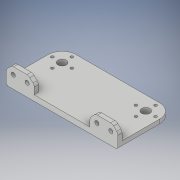
# Autodesk Inventor part: body_v3
Saved by Autodesk Inventor 2019 (Build 230136000, 136)
## iProperties
Created: 2018-12-28
Part Number: body_v3
Material: Generic
Document SubType Name: Modeling
Designer: Daniel
Density: 1 g/cm^3
Appearance: Default
Author: Daniel
Autodesk Inventor part; units mm, degrees
ref_plane "YZ Plane" through (0, 0, 0) normal (1, 0, 0) x (0, 1, 0)
ref_plane "XZ Plane" through (0, 0, 0) normal (0, 1, 0) x (-1, 0, 0)
ref_plane "XY Plane" through (0, 0, 0) normal (0, 0, 1) x (1, 0, 0)
sketch "Sketch1" plane through (0, 0, 0) normal (0, 1, 0) x (-1, 0, 0)
  line L0 (56, 0) -> (-56, 0) projected
  line L1 (0, -49) -> (0, 49) projected
  line L2 (40, -20) -> (-40, -20)
  line L3 (-40, -20) -> (-40, 20)
  line L4 (-40, 20) -> (40, 20)
  line L5 (40, 20) -> (40, -20)
  line L6 (27.5, -35) -> (-27.5, -35) construction
  line L7 (-27.5, -35) -> (-27.5, 35) construction
  line L8 (-27.5, 35) -> (27.5, 35) construction
  line L9 (27.5, 35) -> (27.5, -35) construction
  point P0 (0, 0)
  dimension "d0" = 80
  dimension "d1" = 40
  dimension "d2" = 70
  dimension "d3" = 55
  constraints: 16 end point, 4 parallel, 2 horizontal, 2 perpendicular, 4 other
  measures "d0" distance between parallel lines of L3 L5
  measures "d1" distance between parallel lines of L4 L2
  measures "d2" distance between parallel lines of L8 L6
  measures "d3" distance between parallel lines of L9 L7
extrude "Extrusion1" add sketch "Sketch1" along normal blind 4
sketch "Sketch18" plane through (0, 4, 0) normal (0, 1, 0) x (1, 0, 0)
  line L0 (40, 20) -> (-40, 20) projected
  line L1 (-40, 20) -> (-40, -20) projected
  line L2 (-40, -20) -> (40, -20) projected
  line L3 (40, -20) -> (40, 20) projected
  line L4 (-40, -20) -> (40, -20)
  line L5 (40, -20) -> (40, -17)
  line L6 (40, -17) -> (-40, -17)
  line L7 (-40, -17) -> (-40, -20)
  line L8 (-40, 20) -> (-40, -20) projected
  line L9 (40, -20) -> (40, 20) projected
  line L10 (-40, -20) -> (40, -20) projected
  point P0 (0, 0)
  dimension "d207" = 3
  constraints: 8 end point, 3 collinear, 2 parallel, 1 horizontal, 1 perpendicular
  measures "d207" distance between parallel lines of L6 L4
extrude "Extrusion13" add sketch "Sketch18" along normal blind 10 contours L3 L2 L1 L6
sketch "Sketch19" plane through (0, 4, 0) normal (0, 1, 0) x (1, 0, 0)
  line L0 (-40, -17) -> (40, -17) projected
  line L1 (40, -17) -> (40, 20) projected
  line L2 (40, 20) -> (-40, 20) projected
  line L3 (-40, 20) -> (-40, -17) projected
  line L4 (0, 28) -> (0, -28) projected
  point P0 (0, 0)
  point P1 (-30, 10)
  point P2 (30, 10)
  dimension "d210" = 10
  dimension "d211" = 10
  constraints: 1 symmetric about line
  measures "d210" distance from line of L3 point (-30, 10)
  measures "d211" distance from line of L2 point (-30, 10)
hole "Hole9" at (-30, 4, -10) at (30, 4, -10) direction (0, -1, 0) diameter 6 end through all
sketch "Sketch20" plane through (0, 4, 0) normal (0, 1, 0) x (1, 0, 0)
  circle A0 centre (-30, 10) radius 3 projected
  line L0 (-40, -17) -> (40, -17) projected
  line L1 (40, -17) -> (40, 20) projected
  line L2 (40, 20) -> (-40, 20) projected
  line L3 (-40, 20) -> (-40, -17) projected
  line L4 (-30, -17) -> (-30, 20) construction
  line L5 (-40, 20) -> (-40, -17) projected
  line L6 (40, 20) -> (-40, 20) projected
  line L7 (40, -17) -> (-40, -17) projected
  line L8 (-39.3154, 10) -> (-16.7888, 10) construction
  line L9 (0, 28) -> (0, -28) projected
  point P0 (0, 0)
  point P1 (-37, 10)
  point P2 (-23, 10)
  point P3 (-30, 3)
  point P4 (-30, 17)
  point P5 (37, 10)
  point P6 (23, 10)
  point P7 (30, 3)
  point P8 (30, 17)
  dimension "d219" = 7
  dimension "d220" = 7
  dimension "d221" = 7
  dimension "d222" = 7
  constraints: 8 point on line, 4 end point, 4 symmetric about line, 1 horizontal, 1 parallel, 1 vertical
  measures "d219" distance of A0.centre point (-30, 3)
  measures "d220" distance of A0.centre point (-37, 10)
  measures "d221" distance of A0.centre point (-30, 17)
  measures "d222" distance of A0.centre point (-23, 10)
hole "Hole10" at (-37, 4, -10) at (-23, 4, -10) at (-30, 4, -3) at (-30, 4, -17) at (30, 4, -3) at (37, 4, -10) at (30, 4, -17) at (23, 4, -10) direction (0, -1, 0) diameter 2 end through all
fillet "Fillet11" radius 10 2 edges at (40, 2, -20) (-40, 2, -20)
sketch "Sketch21" plane through (40, 4, 17) normal (0, 0, -1) x (-1, 0, 0)
  line L0 (80, 0) -> (0, 0) projected
  line L1 (80, 0) -> (80, 10) projected
  line L2 (0, 10) -> (80, 10) projected
  line L3 (0, 0) -> (0, 10) projected
  point P0 (40, -4)
  point P1 (5, 5)
  point P2 (75, 5)
  dimension "d232" = 5
  dimension "d233" = 5
  dimension "d234" = 5
  dimension "d235" = 5
  measures "d232" distance from line of L3 point (5, 5)
  measures "d233" distance from line of L2 point (5, 5)
  measures "d234" distance from line of L2 point (75, 5)
  measures "d235" distance from line of L1 point (75, 5)
hole "Hole11" at (35, 9, 17) at (-35, 9, 17) direction (0, 0, 1) diameter 3 end through all
chamfer "Chamfer5" distance 4 angle 45 2 edges at (-40, 14, 18.5) (40, 14, 18.5)
fillet "Fillet12" radius 3 4 edges at (-36, 14, 18.5) (-40, 10, 18.5) (36, 14, 18.5) (40, 10, 18.5)
sketch "Sketch22" plane through (40, 4, 17) normal (0, 0, -1) x (-1, 0, 0)
  circle A0 centre (5, 5) radius 1.5 projected
  circle A1 centre (75, 5) radius 1.5 projected
  arc A2 (0.8787, 6.8787) -> (0, 4.7574) centre (3, 4.7574) ccw projected
  line L0 (0, 0) -> (0, 4.7574) projected
  line L1 (80, 0) -> (0, 0) projected
  line L2 (80, 0) -> (80, 4.7574) projected
  arc A3 (80, 4.7574) -> (79.1213, 6.8787) centre (77, 4.7574) ccw projected
  line L3 (76.8787, 9.1213) -> (79.1213, 6.8787) projected
  arc A4 (76.8787, 9.1213) -> (74.7574, 10) centre (74.7574, 7) ccw projected
  line L4 (5.2426, 10) -> (74.7574, 10) projected
  arc A5 (5.2426, 10) -> (3.1213, 9.1213) centre (5.2426, 7) ccw projected
  line L5 (0.8787, 6.8787) -> (3.1213, 9.1213) projected
  line L6 (10, 0) -> (70, 0) projected
  line L7 (20, 10) -> (60, 10)
  line L8 (60, 10) -> (60, 0)
  line L9 (60, 0) -> (20, 0)
  line L10 (20, 0) -> (20, 10)
  point P0 (40, -4)
  point P1 (40, 5)
  dimension "d247" = 5
  dimension "d248" = 40
  dimension "d256" = 40
  dimension "d257" = 10
  dimension "d258" = 20
  constraints: 8 end point, 2 parallel, 1 horizontal, 1 perpendicular, 1 point on line
  measures "d247" distance from line of L4 point (40, 5)
  measures "d248" distance from line of L0 point (40, 5)
  measures "d256" distance between parallel lines of L8 L10
  measures "d257" distance between parallel lines of L1 L7
  measures "d258" distance between parallel lines of L0 L10
extrude "Extrusion14" cut sketch "Sketch22" against normal up to next contours L4 L8 L1 L10
chamfer "Chamfer6" distance 4 angle 45 2 edges at (-20, 14, 18.5) (20, 14, 18.5)
fillet "Fillet13" radius 3 4 edges at (-24, 14, 18.5) (-20, 10, 18.5) (24, 14, 18.5) (20, 10, 18.5)
sketch "Sketch23" plane through (40, 4, 17) normal (0, 0, -1) x (-1, 0, 0)
  arc A0 (20, 4.7574) -> (19.1213, 6.8787) centre (17, 4.7574) ccw projected
  line L0 (16.8787, 9.1213) -> (19.1213, 6.8787) projected
  arc A1 (16.8787, 9.1213) -> (14.7574, 10) centre (14.7574, 7) ccw projected
  line L1 (5.2426, 10) -> (14.7574, 10) projected
  arc A2 (5.2426, 10) -> (3.1213, 9.1213) centre (5.2426, 7) ccw projected
  line L2 (0.8787, 6.8787) -> (3.1213, 9.1213) projected
  arc A3 (0.8787, 6.8787) -> (0, 4.7574) centre (3, 4.7574) ccw projected
  line L3 (0, 0) -> (0, 4.7574) projected
  line L4 (20, 0) -> (0, 0) projected
  line L5 (20, 0) -> (20, 4.7574) projected
  circle A4 centre (5, 5) radius 1.5 projected
  arc A5 (60.8787, 6.8787) -> (60, 4.7574) centre (63, 4.7574) ccw projected
  line L6 (60, 4.7574) -> (60, 0) projected
  line L7 (80, 0) -> (60, 0) projected
  line L8 (80, 0) -> (80, 4.7574) projected
  arc A6 (80, 4.7574) -> (79.1213, 6.8787) centre (77, 4.7574) ccw projected
  line L9 (76.8787, 9.1213) -> (79.1213, 6.8787) projected
  arc A7 (76.8787, 9.1213) -> (74.7574, 10) centre (74.7574, 7) ccw projected
  line L10 (65.2426, 10) -> (74.7574, 10) projected
  arc A8 (65.2426, 10) -> (63.1213, 9.1213) centre (65.2426, 7) ccw projected
  line L11 (60.8787, 6.8787) -> (63.1213, 9.1213) projected
  circle A9 centre (75, 5) radius 1.5 projected
  point P0 (40, -4)
  point P1 (15, 5)
  point P2 (65, 5)
  dimension "d265" = 5
  dimension "d266" = 5
  dimension "d267" = 5
  dimension "d268" = 5
  measures "d265" distance from line of L5 point (15, 5)
  measures "d266" distance from line of L1 point (15, 5)
  measures "d267" distance from line of L10 point (65, 5)
  measures "d268" distance from line of L6 point (65, 5)
hole "Hole13" at (25, 9, 17) at (-25, 9, 17) direction (0, 0, 1) diameter 3 end through all
chamfer "Chamfer7" distance 1 angle 45 5 edges at (0, 0, -20) (37.0711, 0, -17.0711) (40, 0, 5) (-37.0711, 0, -17.0711) (-40, 0, 5)
body "Solid1"
